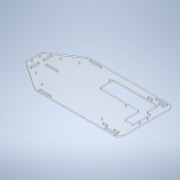
# Autodesk Inventor part: base
Saved by Autodesk Inventor 2020 (Build 240168000, 168)
## iProperties
Created: 2019-09-27
Part Number: base
Material: Polycarbonate, Clear
Document SubType Name: Modeling
Designer: n10208577
Density: 1.2 g/cm^3
Appearance: Polycarbonate - Clear
Author: n10208577
Autodesk Inventor part; units mm, degrees
ref_plane "YZ Plane" through (0, 0, 0) normal (1, 0, 0) x (0, 1, 0)
ref_plane "XZ Plane" through (0, 0, 0) normal (0, 1, 0) x (-1, 0, 0)
ref_plane "XY Plane" through (0, 0, 0) normal (0, 0, 1) x (1, 0, 0)
sketch "Sketch1" plane through (0, 0, 0) normal (0, 1, 0) x (-1, 0, 0)
  line L0 (-100.9651, 48.6333) -> (-100.9651, -1.3667)
  line L1 (79.933, 58.6333) -> (-90.9651, 58.6333)
  line L2 (145.3335, 17.5604) -> (88.3289, 56.0635)
  line L3 (-100.9651, -1.3667) -> (-100.9651, -51.3667)
  circle A0 centre (115.0349, 25.6333) radius 1.6
  circle A1 centre (115.0349, -28.3667) radius 1.6
  circle A2 centre (142.5349, 7.3833) radius 1.6
  circle A3 centre (142.5349, -10.1167) radius 1.6
  circle A4 centre (-94.3651, -9.7667) radius 1.6
  circle A5 centre (-94.3651, 7.0333) radius 1.6
  line L4 (147.5349, -16.1504) -> (147.5349, 13.417)
  arc A6 (-100.9651, -51.3667) -> (-90.9651, -61.3667) centre (-90.9651, -51.3667) ccw
  arc A7 (-90.9651, 58.6333) -> (-100.9651, 48.6333) centre (-90.9651, 48.6333) ccw
  arc A8 (88.3289, 56.0635) -> (79.933, 58.6333) centre (79.933, 43.6333) ccw
  arc A9 (79.933, -61.3667) -> (88.3289, -58.7969) centre (79.933, -46.3667) ccw
  arc A10 (147.5349, 13.417) -> (145.3335, 17.5604) centre (142.5349, 13.417) ccw
  arc A11 (145.3335, -20.2938) -> (147.5349, -16.1504) centre (142.5349, -16.1504) ccw
  line L5 (-90.9651, -61.3667) -> (79.933, -61.3667)
  line L6 (88.3289, -58.7969) -> (145.3335, -20.2938)
  line L7 (-90.9651, -1.3667) -> (-90.9651, 16.6333)
  line L8 (-89.9651, 17.6333) -> (-73.9651, 17.6333)
  arc A12 (-71.9651, 15.6333) -> (-73.9651, 17.6333) centre (-73.9651, 15.6333) ccw
  arc A13 (-89.9651, 17.6333) -> (-90.9651, 16.6333) centre (-89.9651, 16.6333) ccw
  line L9 (-71.9651, 15.6333) -> (-71.9651, -13.3667)
  line L10 (-83.9651, -20.3667) -> (-89.9651, -20.3667)
  arc A14 (-90.9651, -19.3667) -> (-89.9651, -20.3667) centre (-89.9651, -19.3667) ccw
  line L11 (-90.9651, -19.3667) -> (-90.9651, -1.3667)
  line L12 (16.0349, -17.3667) -> (16.0349, -43.3667)
  arc A15 (14.0349, -45.3667) -> (16.0349, -43.3667) centre (14.0349, -43.3667) ccw
  line L13 (14.0349, -15.3667) -> (-69.9651, -15.3667)
  arc A16 (16.0349, -17.3667) -> (14.0349, -15.3667) centre (14.0349, -17.3667) ccw
  arc A17 (-71.9651, -13.3667) -> (-69.9651, -15.3667) centre (-69.9651, -13.3667) ccw
  line L14 (14.0349, -45.3667) -> (-79.9651, -45.3667)
  arc A18 (-81.9651, -43.3667) -> (-79.9651, -45.3667) centre (-79.9651, -43.3667) ccw
  line L15 (-81.9651, -43.3667) -> (-81.9651, -22.3667)
  arc A19 (-81.9651, -22.3667) -> (-83.9651, -20.3667) centre (-83.9651, -22.3667) ccw
  line L16 (-54.6151, -49.4667) -> (-64.3151, -49.4667)
  line L17 (-64.3151, -49.4667) -> (-64.3151, -52.2667)
  line L18 (-59.4651, -52.2667) -> (-54.6151, -52.2667)
  line L19 (-54.6151, -52.2667) -> (-54.6151, -49.4667)
  line L20 (-59.4651, -52.2667) -> (-64.3151, -52.2667)
  line L21 (-79.6151, -49.4667) -> (-89.3151, -49.4667)
  line L22 (-89.3151, -49.4667) -> (-89.3151, -52.2667)
  line L23 (-84.4651, -52.2667) -> (-79.6151, -52.2667)
  line L24 (-79.6151, -52.2667) -> (-79.6151, -49.4667)
  line L25 (-84.4651, -52.2667) -> (-89.3151, -52.2667)
  line L26 (-54.6151, 46.7333) -> (-64.3151, 46.7333)
  line L27 (-64.3151, 46.7333) -> (-64.3151, 49.5333)
  line L28 (-59.4651, 49.5333) -> (-54.6151, 49.5333)
  line L29 (-54.6151, 49.5333) -> (-54.6151, 46.7333)
  line L30 (-59.4651, 49.5333) -> (-64.3151, 49.5333)
  line L31 (-79.6151, 46.7333) -> (-89.3151, 46.7333)
  line L32 (-89.3151, 46.7333) -> (-89.3151, 49.5333)
  line L33 (-84.4651, 49.5333) -> (-79.6151, 49.5333)
  line L34 (-79.6151, 49.5333) -> (-79.6151, 46.7333)
  line L35 (-84.4651, 49.5333) -> (-89.3151, 49.5333)
  circle A20 centre (-45.4651, -11.3667) radius 1.6
  circle A21 centre (-45.4651, 40.6333) radius 1.6
  circle A22 centre (86.5349, 40.6333) radius 1.6
  circle A23 centre (20.0349, -41.3667) radius 1.6
  circle A24 centre (86.5349, -41.3667) radius 1.6
  line L36 (129.6349, -6.5167) -> (129.6349, -24.2167)
  line L37 (132.4349, -6.5167) -> (132.4349, -24.2167)
  line L38 (129.6349, 3.7833) -> (129.6349, 21.4833)
  line L39 (132.4349, 3.7833) -> (132.4349, 21.4833)
  line L40 (119.3849, -2.7667) -> (94.6849, -2.7667)
  line L41 (94.6849, 0.0333) -> (119.3849, 0.0333)
  line L42 (94.6849, 0.0333) -> (94.6849, -2.7667)
  line L43 (119.3849, 0.0333) -> (119.3849, -2.7667)
  line L44 (129.6349, -6.5167) -> (132.4349, -6.5167)
  line L45 (132.4349, -24.2167) -> (129.6349, -24.2167)
  line L46 (129.6349, 3.7833) -> (132.4349, 3.7833)
  line L47 (129.6349, 21.4833) -> (132.4349, 21.4833)
  line L48 (-90.8151, -58.2667) -> (-66.1151, -58.2667)
  line L49 (-66.1151, -58.2667) -> (-66.1151, -55.4667)
  line L50 (-66.1151, -55.4667) -> (-90.8151, -55.4667)
  line L51 (-90.8151, -55.4667) -> (-90.8151, -58.2667)
  line L52 (-90.8151, 55.5333) -> (-66.1151, 55.5333)
  line L53 (-66.1151, 55.5333) -> (-66.1151, 52.7333)
  line L54 (-66.1151, 52.7333) -> (-90.8151, 52.7333)
  line L55 (-90.8151, 52.7333) -> (-90.8151, 55.5333)
  line L56 (54.1849, 55.5333) -> (78.8849, 55.5333)
  line L57 (78.8849, 55.5333) -> (78.8849, 52.7333)
  line L58 (78.8849, 52.7333) -> (54.1849, 52.7333)
  line L59 (54.1849, 52.7333) -> (54.1849, 55.5333)
  line L60 (54.1849, -58.2667) -> (78.8849, -58.2667)
  line L61 (78.8849, -58.2667) -> (78.8849, -55.4667)
  line L62 (78.8849, -55.4667) -> (54.1849, -55.4667)
  line L63 (54.1849, -55.4667) -> (54.1849, -58.2667)
  constraints: 128 end point, 28 point on circle, 25 centre point
extrude "Extrusion1" add sketch "Sketch1" along normal blind 3
body "Solid1"
